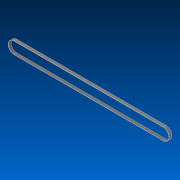
# Autodesk Inventor part: 120T x 9mm Wide Timing Belt (HTD 5mm)(217-3461)
Saved by Autodesk Inventor 2022.2 (Build 262287000, 287)
## iProperties
Created: 2022-01-07
Part Number: 120T x 9mm Wide Timing Belt (HTD 5mm)(217-3461)
Material: Fiberglass Batt
Document SubType Name: Modeling
Designer: omard
Density: 0.032 g/cm^3
Appearance: Gray
Author: omard
Autodesk Inventor part; units mm, degrees
ref_plane "YZ Plane" through (0, 0, 0) normal (1, 0, 0) x (0, 1, 0)
ref_plane "XZ Plane" through (0, 0, 0) normal (0, 1, 0) x (-1, 0, 0)
ref_plane "XY Plane" through (0, 0, 0) normal (0, 0, 1) x (1, 0, 0)
sketch "Sketch1" plane through (0, 0, 0) normal (0, 0, 1) x (1, 0, 0)
  arc A0 (0, 19.1008) -> (0, -19.1008) centre (0, 0) ccw
  arc A1 (495.3, -19.1008) -> (495.3, 19.1008) centre (495.3, 0) ccw
  line L0 (0, 19.1008) -> (495.3, 19.1008)
  line L1 (495.3, -19.1008) -> (0, -19.1008)
  line L2 (495.3, 20.1008) -> (0, 20.1008)
  arc A2 (0, 20.1008) -> (0, -20.1008) centre (0, 0) ccw
  line L3 (0, -20.1008) -> (495.3, -20.1008)
  arc A3 (495.3, -20.1008) -> (495.3, 20.1008) centre (495.3, 0) ccw
  dimension "d0" = 495.3
  dimension "d1" = 38.2016
  dimension "d2" = 1
  constraints: 8 end point, 8 point on circle, 4 centre point, 4 tangent, 1 coincident, 1 equal radius, 1 horizontal alignment, 3 other
  measures "d0" distance of A1.centre point (0, 0)
  measures "d1" diameter of A1
  measures "d2" distance between parallel lines of L0 L2
extrude "Extrusion1" add sketch "Sketch1" along normal mid plane 9
body "Solid1"
